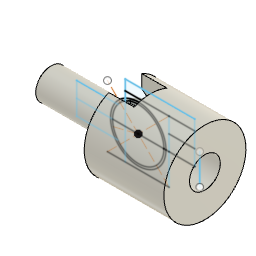
はめ込みジョイント v0 (Autodesk Fusion 360 design; units mm, degrees)
Autodesk Fusion 360 part; units mm, degrees
note: some values were not read from the file. Set by a fixed rule: which face or edge a step refers to.
sketch "スケッチ1" plane through (0, 0, 0) normal (0, 1, 0) x (1, 0, 0)
  circle A0 centre (0, 0) radius 2.5
  line L0 (0, 0) -> (2.5, 0)
  line L1 (0, 0) -> (-2.5, 0)
  line L2 (-6, 1.5) -> (-6, -1.5)
  line L3 (-6, -1.5) -> (-2, -1.5)
  line L4 (6, -1.5) -> (6, 1.5)
  line L5 (-2, 1.5) -> (-6, 1.5)
  line L6 (-2.4254, 0.6063) -> (0, 0) construction
  line L7 (-2.5, 0) -> (-6, 0)
  circle A1 centre (0, 0) radius 2.7
  line L8 (-3, 3) -> (3, 3)
  line L9 (3, 3) -> (3, -3)
  line L10 (3, -3) -> (-1.2688, -3)
  line L11 (-3, 3) -> (3, -3) construction
  line L12 (3, 3) -> (-3, -3) construction
  line L13 (-1.2688, -2.3833) -> (-1.2688, -3)
  line L14 (-1.2688, -2.3833) -> (-1.2688, 3)
  line L15 (3, -3) -> (5.5, -3)
  line L16 (5.5, -3) -> (5.5, 0)
  line L17 (5.5, 0) -> (3, 0)
  line L18 (5.5, -1.5) -> (3, -1.5)
  line L19 (2.5, 0) -> (3, 0)
  line L20 (-1.2688, -3) -> (-1.2688, -4)
  line L21 (-1.2688, -4) -> (5.5, -4)
  line L22 (5.5, -4) -> (5.5, -3)
  dimension "d1" = 5
  dimension "d2" = 12
  dimension "d3" = 3
  dimension "d9" = 5.4
  dimension "d10" = 6
  dimension "d11" = 6
  constraint coincident A0.centre L0.start
  constraint coincident A0 L0.end
  constraint horizontal L0
  constraint coincident A0 L1.end
  constraint parallel L0 L1
  constraint parallel L2 L4
  constraint coincident A0.centre L6
  constraint coincident A0 L3.end
  constraint coincident A0 L5.start
  constraint coincident A0 L6.start
  constraint midpoint L2 L7.end
  constraint perpendicular L2 L7
  constraint horizontal L8
  constraint perpendicular L8 L9
  constraint parallel L8 L10
  constraint coincident L11 A0.centre
  constraint coincident L12 A0.centre
  constraint coincident A1 L13.start
  constraint perpendicular L10 L13
  constraint coincident L8 L14.end
  constraint perpendicular L8 L14
  constraint perpendicular L9 L15
  constraint perpendicular L15 L16
  constraint midpoint L9 L17.end
  constraint perpendicular L9 L17
  constraint midpoint L16 L18.start
  constraint coincident L9 L18.end
  constraint perpendicular L9 L18
  constraint perpendicular L9 L19
  constraint perpendicular L10 L20
  constraint perpendicular L20 L21
  measures "d1" diameter of A0
  measures "d2" distance of L2.end L4.start
  measures "d3" distance of L2.start L2.end
  measures "d9" diameter of A1
  measures "d10" distance of L9.end L12.end
  measures "d11" distance of L8.end L9.end
revolve "回転1" add sketch "スケッチ1" angle 360 about axis through (0, 0, 0) along (1, 0, 0) contours A0 L1 L14 | A0 L3 L7 A1 | A0 L0 L1 L14 | L2 L3 L7 A1 picked at (-2.0827, -0.107) picked at (-0.8459, -0.718) makes body 1
move_face "面を移動1" by (-2.5, 0, 0) 1 faces at (-6, -0.1329, -0.4478) on bodies 1
sketch "スケッチ2" plane through (0, 0, 0) normal (0, 0, 1) x (1, 0, 0)
  line L0 (6, -0.25) -> (-1, -0.25)
  line L1 (-1, -0.25) -> (-1, 0.25)
  line L2 (-1, 0.25) -> (6, 0.25)
  line L3 (6, 0.25) -> (6, -0.25)
  line L4 (6, -0.25) -> (-1, 0.25) construction
  line L5 (-1, -0.25) -> (6, 0.25) construction
  point P0 (2.5, 0)
  dimension "d5" = 7
  dimension "d6" = 0.5
  constraint horizontal L0
  constraint perpendicular L0 L1
  constraint parallel L0 L2
  constraint parallel L1 L3
  constraint coincident L4 P0
  constraint coincident L5 P0
  measures "d5" distance of L1.end L2.end
  measures "d6" distance of L0.end L1.end
extrude "押し出し1" cut sketch "スケッチ2" along normal mid plane 10 bodies 1
revolve "回転2" add sketch "スケッチ1" angle 360 about axis through (5.5, 0, 0) along (-1, 0, 0) separate body contours A1 L9 L10 L13 L19 | L10 L15 L20 L21 L22 | L9 L15 L16 L18 makes body 2
sketch "スケッチ3" plane through (0, 0, 0) normal (0, 0, 1) x (1, 0, 0)
  line L0 (1.2, -1.6) -> (-3.8, -1.6)
  line L1 (-3.8, -1.6) -> (-3.8, 1.6)
  line L2 (-3.8, 1.6) -> (1.2, 1.6)
  line L3 (1.2, 1.6) -> (1.2, -1.6)
  line L4 (1.2, -1.6) -> (-3.8, 1.6) construction
  line L5 (-3.8, -1.6) -> (1.2, 1.6) construction
  point P0 (-1.3, 0)
  dimension "d13" = 5
  dimension "d14" = 3.2
  constraint horizontal L0
  constraint perpendicular L0 L1
  constraint parallel L0 L2
  constraint parallel L1 L3
  constraint coincident L4 P0
  constraint coincident L5 P0
  measures "d13" distance of L1.end L2.end
  measures "d14" distance of L0.end L1.end
extrude "押し出し2" cut sketch "スケッチ3" along normal mid plane 8 bodies 2
move_face "面を移動2" to x (1, 0, 0) y (0, 1, 0) z (0, 0, 1) at (1, 0, 0) 3 faces at (3, 0.1329, -0.4478) (5.5, -0.1828, 3.6621) (5.5, -0.2236, 2.4832) on bodies 2
chamfer "面取り1" distance 0.5 angle 45 2 edges at (-1.2688, 2.3833, 0) (-1.2688, -2.3833, 0) on bodies 2
named bodies: "001", "002"
